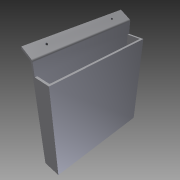
# Autodesk Inventor part: slideFeeder
Saved by Autodesk Inventor 2011 SP1 (Build 150282100, 282)
## iProperties
Created: 2013-01-18
Part Number: slideFeeder
Document SubType Name: Modeling
Designer: wes
Density: 1 g/cm^3
Author: wes
Autodesk Inventor part; units mm, degrees
ref_plane "YZ Plane" through (0, 0, 0) normal (1, 0, 0) x (0, 1, 0)
ref_plane "XZ Plane" through (0, 0, 0) normal (0, 1, 0) x (-1, 0, 0)
sketch "Sketch1" plane through (0, 0, 0) normal (0, 0, 1) x (1, 0, 0)
  line L0 (-19.508, -285.2191) -> (-19.508, 19.5809)
  line L1 (-19.508, 19.5809) -> (-52.5036, 38.6309)
  line L2 (-52.5036, 38.6309) -> (-55.6786, 33.1316)
  line L3 (-19.508, 19.5809) -> (-25.858, 15.9147)
  line L4 (-55.6786, 33.1316) -> (-25.858, 15.9147)
  line L5 (-25.858, 15.9147) -> (-25.858, -285.2191)
  line L6 (-25.858, -285.2191) -> (-19.508, -285.2191)
  point P0 (0, 0)
  dimension "d0" = 120
  dimension "d1" = 304.8
  dimension "d2" = 38.1
  dimension "d4" = 6.35
  constraints: 14 end point, 3 perpendicular, 1 parallel, 1 vertical
  measures "d0" angle of L0 L1
  measures "d1" distance of L0.start L0.end
  measures "d2" distance of L0.end L1.end
  measures "d4" distance between parallel lines of L1 L4
extrude "Extrusion1" add sketch "Sketch1" against normal blind 304.8
fillet "Fillet1" radius 6.35 2 edges at (-19.508, 19.5809, -152.4) (-25.858, 15.9147, -152.4)
sketch "Sketch2" plane through (-52.5036, 38.6309, 0) normal (0.5, 0.8660254, 0) x (0.8660254, -0.5, 0)
  line L0 (0, 0) -> (0, 304.8) projected
  line L1 (34.4338, 0) -> (0, 0) projected
  point P0 (64.7849, 0)
  point P1 (15.24, 50.8)
  point P2 (15.24, 254)
  dimension "d8" = 50.8
  dimension "d10" = 254
  dimension "d11" = 15.24
  dimension "d12" = 15.24
  measures "d8" distance from line of L1 point (15.24, 50.8)
  measures "d10" distance from line of point (15.24, 254) L1
  measures "d11" distance from line of point (15.24, 50.8) L0
  measures "d12" distance from line of L0 point (15.24, 254)
hole "Hole1" at (-39.3054, 31.0109, -50.8) at (-39.3054, 31.0109, -254) direction (-0.5, -0.8660254, 0) diameter 6.858 depth 25.4 tip angle 118
sketch "Sketch3" plane through (-25.858, -285.2191, 0) normal (0, -1, 0) x (1, 0, 0)
  line L0 (0, -304.8) -> (6.35, -304.8) projected
  line L1 (6.35, 0) -> (6.35, -304.8) projected
  line L2 (0, 0) -> (6.35, 0) projected
  line L3 (0, 0) -> (0, -304.8) projected
  line L4 (6.35, 0) -> (52.6401, 0)
  line L5 (52.6401, 0) -> (52.6401, -304.8)
  line L6 (52.6401, -304.8) -> (6.35, -304.8)
  line L7 (6.35, -304.8) -> (6.35, 0)
  line L8 (6.35, -6.35) -> (46.2901, -6.35)
  line L9 (46.2901, -6.35) -> (46.2901, -298.45)
  line L10 (46.2901, -298.45) -> (6.35, -298.45)
  line L11 (6.35, -298.45) -> (6.35, -6.35)
  point P0 (25.858, 0)
  dimension "d20" = 6.35
  dimension "d21" = 6.35
  dimension "d22" = 6.35
  constraints: 16 end point, 4 parallel, 2 horizontal, 2 perpendicular, 1 point on line
  measures "d20" distance between parallel lines of L5 L9
  measures "d21" distance between parallel lines of L4 L8
  measures "d22" distance between parallel lines of L10 L6
ref_plane "Work Plane1" through (-22.683, 21.414, 0) normal (0.5, 0.8660254, 0) x (-0.8660254, 0.5, 0)
extrude "Extrusion2" add sketch "Sketch3" against normal blind 266.7 contours L1 L10 L9 L8 L4 L5 L6
thread "Thread1" size "5/16-18 UNC" class "2B" standard "ANSI Unified Screw Threads" full length
thread "Thread2" size "5/16-18 UNC" class "2B" standard "ANSI Unified Screw Threads" full length
body "Solid1"
